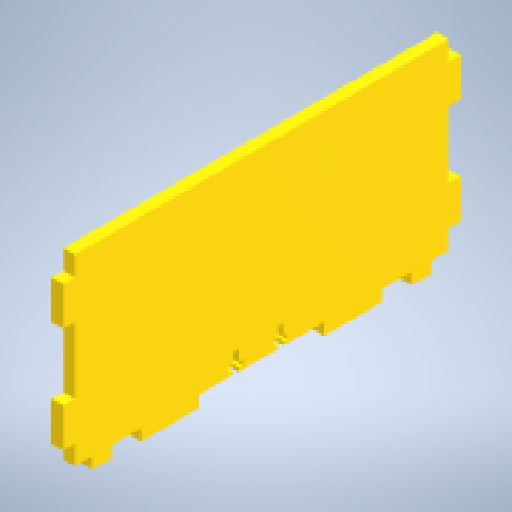
# Autodesk Inventor part: перед
Saved by Autodesk Inventor 2024.2 (Build 282272000, 272)
## iProperties
Created: 2026-01-28
Part Number: перед
Material: Типовые
Document SubType Name: Modeling
Designer: Zakhar
Density: 1 g/cm^3
Appearance: Глянцевая — золотая
Author: Zakhar
Autodesk Inventor part; units mm, degrees
ref_plane "YZ Plane" through (0, 0, 0) normal (1, 0, 0) x (0, 1, 0)
ref_plane "XZ Plane" through (0, 0, 0) normal (0, 1, 0) x (-1, 0, 0)
ref_plane "XY Plane" through (0, 0, 0) normal (0, 0, 1) x (1, 0, 0)
sketch "Эскиз1" plane through (0, 0, 0) normal (1, 0, 0) x (0, 1, 0)
  line L0 (97.2644, 106.089) -> (-2.7356, 106.089)
  line L1 (-2.7356, 106.089) -> (-2.7356, -97.911)
  line L2 (-2.7356, -97.911) -> (97.2644, -97.911)
  line L3 (97.2644, -97.911) -> (97.2644, 106.089)
  line L4 (-2.7356, 106.089) -> (3.2644, 106.089)
  line L5 (3.2644, 106.089) -> (3.2644, 66.089)
  line L6 (3.2644, 66.089) -> (-2.7356, 66.089)
  line L7 (-2.7356, 66.089) -> (-2.7356, 106.089)
  line L8 (3.2644, 66.089) -> (-2.7356, 66.089)
  line L9 (-2.7356, 66.089) -> (-2.7356, 36.089)
  line L10 (-2.7356, 36.089) -> (3.2644, 36.089)
  line L11 (3.2644, 36.089) -> (3.2644, 66.089)
  line L12 (-2.7356, 36.089) -> (3.2644, 36.089)
  line L13 (3.2644, 36.089) -> (3.2644, -27.911)
  line L14 (3.2644, -27.911) -> (-2.7356, -27.911)
  line L15 (-2.7356, -27.911) -> (-2.7356, 36.089)
  line L16 (3.2644, -27.911) -> (-2.7356, -27.911)
  line L17 (-2.7356, -27.911) -> (-2.7356, -57.911)
  line L18 (-2.7356, -57.911) -> (3.2644, -57.911)
  line L19 (3.2644, -57.911) -> (3.2644, -27.911)
  line L20 (3.2644, -57.911) -> (-2.7356, -57.911)
  line L21 (-2.7356, -57.911) -> (-2.7356, -97.911)
  line L22 (-2.7356, -97.911) -> (3.2644, -97.911)
  line L23 (3.2644, -97.911) -> (3.2644, -57.911)
  line L24 (3.2644, 91.089) -> (-2.7356, 91.089)
  line L25 (-2.7356, 91.089) -> (-2.7356, 81.089)
  line L26 (-2.7356, 81.089) -> (3.2644, 81.089)
  line L27 (3.2644, 81.089) -> (3.2644, 91.089)
  line L28 (3.2644, -72.911) -> (-2.7356, -72.911)
  line L29 (-2.7356, -72.911) -> (-2.7356, -82.911)
  line L30 (-2.7356, -82.911) -> (3.2644, -82.911)
  line L31 (3.2644, -82.911) -> (3.2644, -72.911)
  point P0 (0, 0)
  point P1 (-2.7356, 66.089)
  point P2 (3.2644, 36.089)
  point P3 (-2.7356, -27.911)
  point P4 (0.2644, 91.089)
  point P5 (0.2644, 81.089)
  point P6 (0.2644, 66.089)
  point P7 (0.2644, -57.911)
  point P8 (0.2644, -72.911)
  point P9 (0.2644, -82.911)
  dimension "d0" = 204
  dimension "d1" = 100
  dimension "d2" = 40
  dimension "d3" = 30
  dimension "d4" = 30
  dimension "d5" = 40
  dimension "d8" = 6
  dimension "d41" = 10
  dimension "d42" = 15
  dimension "d43" = 15
  dimension "d44" = 10
  constraints: 64 end point, 16 parallel, 8 horizontal, 8 perpendicular, 7 point on line, 6 midpoint
  measures "d0" distance of L0.end L1.end
  measures "d1" distance of L0.start L0.end
  measures "d2" distance of L4.end L5.end
  measures "d3" distance of L10.end L5.end
  measures "d4" distance of L18.end L13.end
  measures "d5" distance of L22.end L18.end
  measures "d8" distance of L5.end L6.end
  measures "d41" distance of point (0.264, 91.089) point (0.264, 81.089)
  measures "d42" distance of point (0.264, 66.089) point (0.264, 81.089)
  measures "d43" distance from line of point (0.264, -57.911) L28
  measures "d44" distance of point (0.264, -72.911) point (0.264, -82.911)
extrude "Выдавливание1" add sketch "Эскиз1" along normal blind 6 contours L3 L2 L23 L19 L13 L11 L5 L0 | L5 L26 L1 L24 | L30 L1 L28 L23 | L11 L10 L1 L6 | L18 L1 L14 L19
sketch "Эскиз2" plane through (6, 0, 0) normal (1, 0, 0) x (0, 0, -1)
  line L0 (-106.089, 97.2644) -> (-106.089, 3.2644) projected
  line L1 (-106.089, 3.2644) -> (-100.089, 3.2644)
  line L2 (-100.089, 3.2644) -> (-100.089, 13.2644)
  line L3 (-100.089, 13.2644) -> (-106.089, 13.2644)
  line L4 (-106.089, 13.2644) -> (-106.089, 3.2644)
  line L5 (-106.089, 33.2644) -> (-100.089, 33.2644)
  line L6 (-100.089, 33.2644) -> (-100.089, 13.2644)
  line L7 (-100.089, 13.2644) -> (-106.089, 13.2644)
  line L8 (-106.089, 13.2644) -> (-106.089, 33.2644)
  line L9 (-100.089, 33.2644) -> (-106.089, 33.2644)
  line L10 (-106.089, 33.2644) -> (-106.089, 67.2644)
  line L11 (-106.089, 67.2644) -> (-100.089, 67.2644)
  line L12 (-100.089, 67.2644) -> (-100.089, 33.2644)
  line L13 (-100.089, 67.2644) -> (-106.089, 67.2644)
  line L14 (-106.089, 67.2644) -> (-106.089, 87.2644)
  line L15 (-106.089, 87.2644) -> (-100.089, 87.2644)
  line L16 (-100.089, 87.2644) -> (-100.089, 67.2644)
  line L17 (-100.089, 87.2644) -> (-106.089, 87.2644)
  line L18 (-106.089, 87.2644) -> (-106.089, 97.2644)
  line L19 (-106.089, 97.2644) -> (-100.089, 97.2644)
  line L20 (-100.089, 97.2644) -> (-100.089, 87.2644)
  line L21 (57.911, 3.2644) -> (97.911, 3.2644) projected
  line L22 (97.911, 3.2644) -> (91.911, 3.2644)
  line L23 (91.911, 3.2644) -> (91.911, 13.2644)
  line L24 (91.911, 13.2644) -> (97.911, 13.2644)
  line L25 (97.911, 13.2644) -> (97.911, 3.2644)
  line L26 (97.911, 13.2644) -> (91.911, 13.2644)
  line L27 (91.911, 13.2644) -> (91.911, 33.2644)
  line L28 (91.911, 33.2644) -> (97.911, 33.2644)
  line L29 (97.911, 33.2644) -> (97.911, 13.2644)
  line L30 (97.911, 33.2644) -> (91.911, 33.2644)
  line L31 (91.911, 33.2644) -> (91.911, 67.2644)
  line L32 (91.911, 67.2644) -> (97.911, 67.2644)
  line L33 (97.911, 67.2644) -> (97.911, 33.2644)
  line L34 (97.911, 67.2644) -> (91.911, 67.2644)
  line L35 (91.911, 67.2644) -> (91.911, 87.2644)
  line L36 (91.911, 87.2644) -> (97.911, 87.2644)
  line L37 (97.911, 87.2644) -> (97.911, 67.2644)
  line L38 (97.911, 87.2644) -> (91.911, 87.2644)
  line L39 (91.911, 87.2644) -> (91.911, 97.2644)
  line L40 (91.911, 97.2644) -> (97.911, 97.2644)
  line L41 (97.911, 97.2644) -> (97.911, 87.2644)
  point P0 (0, 0)
  point P1 (91.911, 3.2644)
  dimension "d9" = 10
  dimension "d10" = 20
  dimension "d11" = 10
  dimension "d12" = 20
  dimension "d13" = 34
  dimension "d14" = 6
  dimension "d15" = 10
  dimension "d16" = 20
  dimension "d17" = 20
  dimension "d18" = 10
  dimension "d19" = 34
  dimension "d20" = 6
  constraints: 80 end point, 20 parallel, 10 horizontal, 10 perpendicular, 8 point on line
  measures "d9" distance of L1.end L2.end
  measures "d10" distance of L5.end L2.end
  measures "d11" distance of L19.end L15.end
  measures "d12" distance of L15.end L11.end
  measures "d13" distance of L11.end L5.end
  measures "d14" distance of L0.end L1.end
  measures "d15" distance of L22.end L23.end
  measures "d16" distance of L26.end L27.end
  measures "d17" distance of L34.end L35.end
  measures "d18" distance of L38.end L39.end
  measures "d19" distance of L30.end L31.end
  measures "d20" distance of L23.end L24.end
extrude "Выдавливание2" cut sketch "Эскиз2" against normal through all contours L19 L20 L15 L0 | L11 L12 L5 L0 | L3 L2 L1 L0 | L23 L24 L25 L21 | L31 L32 L33 L28 | L39 L40 L41 L36
sketch "Эскиз4" plane through (6, 0, 0) normal (1, 0, 0) x (0, 0, -1)
  line L0 (-36.089, 3.2644) -> (27.911, 3.2644) projected
  line L1 (-19, 3.2644) -> (-16, 3.2644)
  line L2 (-16, 3.2644) -> (-16, 13.2644)
  line L3 (-16, 13.2644) -> (-19, 13.2644)
  line L4 (-19, 13.2644) -> (-19, 3.2644)
  line L5 (-21, 7.6644) -> (-14, 7.6644)
  line L6 (-14, 7.6644) -> (-14, 5.2644)
  line L7 (-14, 5.2644) -> (-21, 5.2644)
  line L8 (-21, 5.2644) -> (-21, 7.6644)
  line L9 (7, 3.2644) -> (4, 3.2644)
  line L10 (4, 3.2644) -> (4, 13.2644)
  line L11 (4, 13.2644) -> (7, 13.2644)
  line L12 (7, 13.2644) -> (7, 3.2644)
  line L13 (2, 7.6644) -> (9, 7.6644)
  line L14 (9, 7.6644) -> (9, 5.2644)
  line L15 (9, 5.2644) -> (2, 5.2644)
  line L16 (2, 5.2644) -> (2, 7.6644)
  point P0 (0, 0)
  point P1 (4, 5.2644)
  point P2 (4, 3.2644)
  point P3 (7, 5.2644)
  point P4 (7, 7.6644)
  point P5 (4, 7.6644)
  point P6 (-19, 5.2644)
  point P7 (-16, 3.2644)
  point P8 (-16, 5.2644)
  point P9 (-16, 7.6644)
  point P10 (-19, 7.6644)
  dimension "d26" = 7
  dimension "d27" = 7
  dimension "d28" = 2
  dimension "d29" = 3
  dimension "d30" = 2.4
  dimension "d31" = 10
  dimension "d32" = 16
  dimension "d33" = 2
  dimension "d34" = 2.4
  dimension "d35" = 2
  dimension "d36" = 3
  dimension "d37" = 10
  dimension "d38" = 4
  constraints: 32 end point, 8 parallel, 4 horizontal, 4 perpendicular, 3 point on line
  measures "d26" distance of L14.end L15.end
  measures "d27" distance of L6.end L7.end
  measures "d28" distance between parallel lines of L8 L4
  measures "d29" distance of L2.end L3.end
  measures "d30" distance between parallel lines of L5 L7
  measures "d31" distance of L1.end L2.end
  measures "d32" distance from line of L2 point (0, 0)
  measures "d33" distance between parallel lines of L0 L7
  measures "d34" distance between parallel lines of L15 L13
  measures "d35" distance between parallel lines of L12 L14
  measures "d36" distance of L10.end L11.end
  measures "d37" distance of L11.end L9.start
  measures "d38" distance from line of point (0, 0) L10
extrude "Выдавливание4" cut sketch "Эскиз4" against normal blind 6.25
